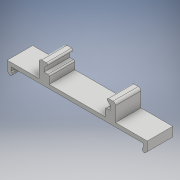
# Autodesk Inventor part: env_combo_holder
Saved by Autodesk Inventor 2018 (Build 220112000, 112)
## iProperties
Created: 2021-06-06
Part Number: env_combo_holder
Material: Generic
Document SubType Name: Modeling
Designer: Kevin
Density: 1 g/cm^3
Appearance: Default
Author: Kevin
Autodesk Inventor part; units mm, degrees
ref_plane "YZ Plane" through (0, 0, 0) normal (1, 0, 0) x (0, 1, 0)
ref_plane "XZ Plane" through (0, 0, 0) normal (0, 1, 0) x (-1, 0, 0)
ref_plane "XY Plane" through (0, 0, 0) normal (0, 0, 1) x (1, 0, 0)
sketch "Sketch1" plane through (0, 0, 0) normal (0, 0, 1) x (1, 0, 0)
  line L0 (-26, 5) -> (26, 5)
  line L1 (26, 5) -> (26, -5)
  line L2 (26, -5) -> (-26, -5)
  line L3 (-26, -5) -> (-26, 5)
  point P0 (0, 0)
  dimension "d0" = 52
  dimension "d1" = 10
  constraints: 8 end point, 2 parallel, 1 horizontal, 1 perpendicular
  measures "d0" distance of L1.end L2.end
  measures "d1" distance of L0.end L1.end
extrude "Extrusion1" add sketch "Sketch1" along normal blind 1.5
sketch "Sketch2" plane through (-26, -5, 0) normal (0, -1, 0) x (1, 0, 0)
  line L0 (0, 1.5) -> (52, 1.5) projected
  line L1 (26, 1.5) -> (13, 1.5)
  line L2 (13, 4.7) -> (15, 4.7)
  line L3 (15, 4.7) -> (15, 1.5)
  line L4 (13, 4.7) -> (13, 6.3)
  line L5 (13, 6.3) -> (15, 8.3)
  line L6 (13, 6.3) -> (15.8284, 6.3) construction
  line L7 (15, 8.3) -> (11, 8.3)
  line L8 (11, 8.3) -> (11, 1.5)
  line L9 (52, 1.5) -> (0, 1.5) projected
  line L10 (11, 1.5) -> (15, 1.5)
  line L11 (26, 1.5) -> (26, 4.9)
  line L12 (39, 4.7) -> (37, 4.7)
  line L13 (37, 4.7) -> (37, 1.5)
  line L14 (39, 4.7) -> (39, 6.3)
  line L15 (39, 6.3) -> (37, 8.3)
  line L16 (39, 6.3) -> (36.1716, 6.3) construction
  line L17 (37, 8.3) -> (41, 8.3)
  line L18 (41, 8.3) -> (41, 1.5)
  line L19 (41, 1.5) -> (37, 1.5)
  point P0 (26, 0)
  point P1 (39, 1.5)
  dimension "d4" = 13
  dimension "d5" = 3.2
  dimension "d6" = 2
  dimension "d7" = 1.6
  dimension "d8" = 45
  constraints: 36 end point, 9 symmetric about line, 3 horizontal, 3 point on line, 2 perpendicular, 2 vertical, 1 collinear, 1 equal length, 1 midpoint
  measures "d4" distance of L1.start L1.end
  measures "d5" distance of L1.end L2.start
  measures "d6" distance of L2.start L2.end
  measures "d7" distance of L2.start L4.end
  measures "d8" angle of L6 L5
extrude "Extrusion2" add sketch "Sketch2" against normal blind 10
sketch "Sketch3" plane through (-26, -5, 0) normal (0, -1, 0) x (1, 0, 0)
  line L0 (0, 0) -> (52, 0) projected
  line L1 (0, 0) -> (0, -1.5)
  line L2 (0, 0) -> (0, 1.5) projected
  line L3 (0, 1.5) -> (-1.5, 1.5)
  line L4 (0, -1.5) -> (0.75, -2.25)
  line L5 (0, -1.5) -> (4.2622, -1.5) construction
  line L6 (0.75, -2.25) -> (-0.3107, -3.3107)
  line L7 (0.75, -2.25) -> (-0.3107, -3.3107)
  line L8 (0, 1.5) -> (-1.5, 1.5)
  line L9 (-1.5, 1.5) -> (-1.5, -2.1213)
  line L10 (-0.3107, -3.3107) -> (-1.5, -2.1213)
  line L11 (26, 0) -> (26, -3.3107)
  line L12 (52, 0) -> (52, -1.5)
  line L13 (52, 0) -> (52, 1.5)
  line L14 (52, 1.5) -> (53.5, 1.5)
  line L15 (52, -1.5) -> (51.25, -2.25)
  line L16 (52, -1.5) -> (47.7378, -1.5) construction
  line L17 (51.25, -2.25) -> (52.3107, -3.3107)
  line L18 (51.25, -2.25) -> (52.3107, -3.3107)
  line L19 (52, 1.5) -> (53.5, 1.5)
  line L20 (53.5, 1.5) -> (53.5, -2.1213)
  line L21 (52.3107, -3.3107) -> (53.5, -2.1213)
  dimension "d11" = 1.5
  dimension "d13" = 45
  dimension "d15" = 1.5
  constraints: 40 end point, 7 symmetric about line, 3 vertical, 2 horizontal, 2 perpendicular
  measures "d11" distance of L0.start L1.end
  measures "d13" angle of L4 L5
  measures "d15" distance of L6.end L4.end
extrude "Extrusion3" add sketch "Sketch3" against normal blind 10
fillet "Fillet1" radius 0.5 4 edges at (-25.25, 0, -2.25) (-26.3107, 0, -3.3107) (25.25, 0, -2.25) (26.3107, 0, -3.3107)
fillet "Fillet2" radius 1 2 edges at (-15, 0, 8.3) (15, 0, 8.3)
fillet "Fillet3" radius 0.5 2 edges at (-11, 0, 8.3) (11, 0, 8.3)
fillet "Fillet4" radius 0.5 2 edges at (-11, 0, 4.7) (11, 0, 4.7)
body "Solid1"
